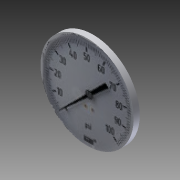
# Autodesk Inventor part: PSI Guage Face 1764
Saved by Autodesk Inventor 2011 (Build 150239000, 239)
## iProperties
Created: 2010-02-12
Part Number: PSI Guage Face 1764
Document SubType Name: Modeling
Designer: jgehrig
Density: 1 g/cm^3
Author: jgehrig
Autodesk Inventor part; units mm, degrees
ref_plane "YZ Plane" through (0, 0, 0) normal (1, 0, 0) x (0, 1, 0)
ref_plane "XZ Plane" through (0, 0, 0) normal (0, 1, 0) x (-1, 0, 0)
ref_plane "XY Plane" through (0, 0, 0) normal (0, 0, 1) x (1, 0, 0)
sketch "Sketch1" plane through (0, 0, 0) normal (0, 0, 1) x (1, 0, 0)
  circle A0 centre (0.6319, 0) radius 19.3675
  point P0 (0, 0)
  dimension "d0" = 38.735
  constraints: 1 centre point
  measures "d0" diameter of A0
extrude "Extrusion1" add sketch "Sketch1" along normal blind 2.54
sketch "Sketch2" plane through (0.6319, 0, 2.54) normal (0, 0, 1) x (1, 0, 0)
  line L0 (-22.6669, 22.0575) -> (22.4736, 22.0575) construction
  line L1 (22.4736, 22.0575) -> (22.4736, -26.3036) construction
  line L2 (22.4736, -26.3036) -> (-22.6669, -26.3036) construction
  line L3 (-22.6669, -26.3036) -> (-22.6669, 22.0575) construction
  point P0 (-0.6319, 0)
  constraints: 2 other
decal "Decal1"
body "Solid1"
